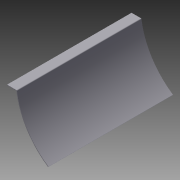
# Autodesk Inventor part: 8 ball ramp
Saved by Autodesk Inventor 2012 (Build 160160000, 160)
## iProperties
Created: 2013-10-24
Part Number: 8 ball ramp
Material: Default
Document SubType Name: Modeling
Designer: Bryce
Density: 1 g/cm^3
Author: Bryce
Autodesk Inventor part; units mm, degrees
ref_plane "YZ Plane" through (0, 0, 0) normal (1, 0, 0) x (0, 1, 0)
ref_plane "XZ Plane" through (0, 0, 0) normal (0, 1, 0) x (-1, 0, 0)
ref_plane "XY Plane" through (0, 0, 0) normal (0, 0, 1) x (1, 0, 0)
sketch "Sketch1" plane through (0, 0, 0) normal (0, 0, 1) x (1, 0, 0)
  line L0 (0, 0) -> (-22.225, 0)
  line L1 (-22.225, 0) -> (-22.225, 1.5875)
  line L2 (-22.225, 1.5875) -> (1.377, 1.5875)
  arc A0 (0, 0) -> (76.2, -120.242) centre (173.0503, 25.4) ccw
  arc A1 (1.377, 1.5875) -> (77.0791, -118.92) centre (173.0503, 25.4) ccw
  line L3 (77.0791, -118.92) -> (76.2, -120.242)
  dimension "d0" = 1.5875
  dimension "d1" = 22.225
  dimension "d2" = 174.9044
  dimension "d3" = 25.4
  dimension "d4" = 76.2
  dimension "d5" = 1.5875
  constraints: 8 end point, 4 point on circle, 2 centre point, 1 coincident, 1 horizontal, 1 parallel, 1 perpendicular, 1 point on line
  measures "d0" distance of L0.end L1.end
  measures "d1" distance of L0.start L0.end
  measures "d2" radius of A0
  measures "d3" distance from line of A0.centre L0
  measures "d4" horizontal distance of L0.start L3.end
  measures "d5" distance of L3.start L3.end
extrude "Extrusion1" add sketch "Sketch1" along normal blind 298.45
fillet "Fillet1" radius 1.5875 1 edges at (1.377, 1.5875, 149.225)
body "Solid1"
